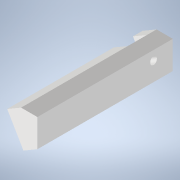
# Autodesk Inventor part: Slider
Saved by Autodesk Inventor 2020 (Build 240168000, 168)
## iProperties
Created: 2020-03-31
Part Number: Slider
Material: Generisch
Document SubType Name: Modeling
Designer: Fynn
Density: 1 g/cm^3
Appearance: Vorgabe
Author: Fynn
Autodesk Inventor part; units mm, degrees
ref_plane "YZ Plane" through (0, 0, 0) normal (1, 0, 0) x (0, 1, 0)
ref_plane "XZ Plane" through (0, 0, 0) normal (0, 1, 0) x (-1, 0, 0)
sketch "Skizze1" plane through (0, 0, 0) normal (0, 0, 1) x (1, 0, 0)
  line L0 (0, 0) -> (-5.0357, 8.6396) projected
  line L1 (-5.0357, 8.6396) -> (-9.3555, 6.1217) projected
  line L2 (-4.3198, -2.5178) -> (-9.3555, 6.1217) projected
  line L3 (0, 0) -> (-4.3198, -2.5178) projected
  line L4 (0, 0) -> (0, 8.6396)
  line L5 (0, 8.6396) -> (-5.0357, 8.6396)
  constraints: 4 end point, 1 perpendicular, 1 vertical
extrude "Extrusion1" add sketch "Skizze1" along normal blind 3
sketch "Skizze2" plane through (0, 0, 3) normal (0, 0, 1) x (1, 0, 0)
  line L0 (0, 8.6396) -> (-5.0357, 8.6396) projected
  line L1 (0, 0) -> (0, 8.6396) projected
  line L2 (-4.3198, -2.5178) -> (0, 0) projected
  line L3 (-9.3555, 6.1217) -> (-4.3198, -2.5178) projected
  line L4 (-5.0357, 8.6396) -> (-9.3555, 6.1217) projected
  line L5 (0, 0) -> (-5.0357, 8.6396) projected
  line L6 (0, 0) -> (-4.3198, -2.5178) projected
  line L7 (-9.3555, 6.1217) -> (-4.3198, -2.5178) projected
  line L8 (-5.0357, 8.6396) -> (-9.3555, 6.1217) projected
ref_plane "Arbeitsebene1" through (-10.5829, -3.5471, -5.9368) normal (0, 0, -1) x (0, 1, 0)
extrude "Extrusion2" add sketch "Skizze2" against normal up to surface (8.9368 mm away) contours L1 L5 L0
sketch "Skizze3" plane through (0, 8.6396, -5.9368) normal (0, 0, -1) x (-1, 0, 0)
  line L0 (6.3089, -7.7448) -> (1.9891, -5.2269)
  line L1 (0, -8.6396) -> (5.0357, 0) projected
  line L2 (0, -8.6396) -> (4.3198, -11.1574) projected
  line L3 (9.3555, -2.5178) -> (4.3198, -11.1574) projected
  line L4 (5.0357, 0) -> (9.3555, -2.5178) projected
  line L5 (0, -8.6396) -> (0, 0) projected
  line L6 (5.0357, 0) -> (0, -8.6396) projected
  line L7 (0, 0) -> (5.0357, 0) projected
  constraints: 2 end point, 3 other
extrude "Extrusion3" add sketch "Skizze3" along normal blind 3
sketch "Skizze4" plane through (-5.0357, 8.6396, -5.9368) normal (-0.8639552, -0.5035686, 0) x (0, 0, 1)
  circle A0 centre (2.9684, -5) radius 1.05 projected
  point P0 (5.9368, -10)
extrude "Extrusion4" cut sketch "Skizze4" against normal through all
sketch "Skizze6" plane through (0, 0, 3) normal (0, 0, 1) x (1, 0, 0)
  line L0 (-5.0357, 8.6396) -> (-9.3555, 6.1217) projected
  line L1 (-9.3555, 6.1217) -> (-4.3198, -2.5178) projected
  line L2 (-4.3198, -2.5178) -> (0, 0) projected
  line L3 (0, 0) -> (0, 8.6396) projected
  line L4 (0, 8.6396) -> (-5.0357, 8.6396) projected
extrude "Extrusion5" add sketch "Skizze6" along normal blind 30
sketch "Skizze7" plane through (0, 0, 33) normal (0, 0, 1) x (1, 0, 0)
  line L0 (0, 8.6396) -> (0, 0) projected
  line L1 (0, 8.6396) -> (-6, 8.6396)
  line L2 (-6, 8.6396) -> (-6, -6.275)
  line L3 (-6, -6.275) -> (0, -6.275)
  line L4 (0, -6.275) -> (0, 8.6396)
  line L5 (-4.3198, -2.5178) -> (0, 0) projected
  line L6 (0, 0) -> (0, 8.6396) projected
  line L7 (0, 8.6396) -> (-5.0357, 8.6396) projected
  line L8 (-5.0357, 8.6396) -> (-9.3555, 6.1217) projected
  line L9 (-9.3555, 6.1217) -> (-4.3198, -2.5178) projected
  point P0 (-6, 0.3649)
  point P1 (-6, 8.0775)
  dimension "d10" = 6
  constraints: 8 end point, 2 parallel, 1 horizontal, 1 perpendicular
  measures "d10" distance between parallel lines of L2 L0
extrude "Extrusion6" cut sketch "Skizze7" against normal blind 30 contours L2 L9 L8
sketch "Skizze8" plane through (-6, 0.3649, 33) normal (-1, 0, 0) x (0, 0, 1)
  line L0 (-3.2, 3.2747) -> (-25.8, 3.2747) construction
  line L1 (-3.2, 4.4747) -> (-25.8, 4.4747)
  line L2 (-25.8, 2.0747) -> (-3.2, 2.0747)
  arc A0 (-3.2, 2.0747) -> (-3.2, 4.4747) centre (-3.2, 3.2747) ccw
  arc A1 (-25.8, 4.4747) -> (-25.8, 2.0747) centre (-25.8, 3.2747) ccw
  line L3 (0, 7.7126) -> (0, 0) projected
  line L4 (-33, 8.2747) -> (0, 8.2747) projected
  point P0 (-33, -0.3649)
  point P1 (-14.5, 3.2747)
  dimension "d13" = 2.4
  dimension "d14" = 25
  dimension "d15" = 2
  dimension "d16" = 5
  constraints: 8 end point, 4 point on circle, 4 tangent, 2 centre point, 1 horizontal, 1 midpoint, 1 parallel
  measures "d13" diameter of A1
  measures "d15" distance edge to line of A0 L3
  measures "d16" distance from line of L4 point (-14.5, 3.275)
extrude "Extrusion7" cut sketch "Skizze8" against normal blind 30
ref_plane "Arbeitsebene2" through (0, 8.6396, -8.9368) normal (-0.8639552, -0.5035686, 0) x (0, 0, 1)
sketch "Skizze9" plane through (0, 8.6396, -8.9368) normal (-0.8639552, -0.5035686, 0) x (0, 0, 1)
  circle A0 centre (5.9684, -2.4642) radius 1.05 projected
  circle A1 centre (5.9684, -2.4642) radius 1.05 projected
  circle A2 centre (5.9684, -2.4642) radius 2.2
  point P0 (8.9368, -7.4642)
  dimension "d19" = 4.4
  constraints: 1 centre point, 1 coincident
  measures "d19" diameter of A2
extrude "Extrusion8" cut sketch "Skizze9" along normal blind 2
sketch "Skizze10" plane through (0, 0, 0) normal (0, 0, -1) x (-1, 0, 0)
  line L0 (5.0357, 8.6396) -> (0, 0) projected
  line L1 (4.3198, -2.5178) -> (0, 0) projected
  line L2 (9.3555, 6.1217) -> (4.3198, -2.5178) projected
  line L3 (5.0357, 8.6396) -> (9.3555, 6.1217) projected
extrude "Extrusion9" cut sketch "Skizze10" along normal blind 6.5 and the other way blind 0.5
